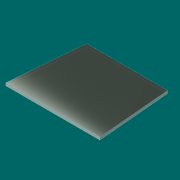
# Autodesk Inventor part: mirrorTopBottom
Saved by Autodesk Inventor 2016 (Build 200138000, 138)
## iProperties
Created: 2015-10-14
Part Number: mirrorTopBottom
Material: Glass
Document SubType Name: Modeling
Designer: Sawaiz
Density: 2.18 g/cm^3
Appearance: Clear
Author: Sawaiz
Autodesk Inventor part; units mm, degrees
ref_plane "YZ Plane" through (0, 0, 0) normal (1, 0, 0) x (0, 1, 0)
ref_plane "XZ Plane" through (0, 0, 0) normal (0, 1, 0) x (-1, 0, 0)
ref_plane "XY Plane" through (0, 0, 0) normal (0, 0, 1) x (1, 0, 0)
sketch "Sketch1" plane through (0, 0, 0) normal (0, 0, 1) x (1, 0, 0)
  line L0 (-37.1597, -43.7763) -> (-37.1597, 43.7763)
  line L1 (-37.1597, 43.7763) -> (43.1218, 50.8)
  line L2 (43.1218, 50.8) -> (43.1218, -50.8)
  line L3 (43.1218, -50.8) -> (-37.1597, -43.7763)
  line L4 (-37.1597, -43.7763) -> (43.1218, 50.8) construction
  line L5 (-37.1597, 43.7763) -> (43.1218, -50.8) construction
  point P0 (0, 0)
  dimension "d0" = 85
  dimension "d1" = 101.6
  dimension "d2" = 80.2815
  dimension "d5" = 87.5526
  constraints: 12 end point, 2 point on line, 1 equal length, 1 parallel, 1 vertical
  measures "d0" angle of L2 L1
  measures "d1" distance of L1.end L2.end
  measures "d2" distance between parallel lines of L2 L0
  measures "d5" distance of L0.start L0.end
extrude "Extrusion1" add sketch "Sketch1" along normal blind 3
equation "\"d1\" = width"
equation "\"d3\" = mirrorThickness"
equation "\"acrylicThickness\" = 6.35"
equation "\"height\" = 101.6"
equation "\"width\" = 101.6"
equation "\"depth\" = 101.6"
equation "\"mirrorAngle\" = 5deg"
equation "\"detectorWidth\" = 52"
equation "\"detectorHeight\" = 52"
equation "\"mirrorThickness\" = 3"
equation "\"fresnelThickness\" = 0.1"
equation "\"focalLength\" = 76.2"
equation "\"ior\" = 1.49"
equation "\"centerThickness\" = 1.524"
equation "\"fresnelAngle\" = 90deg"
equation "\"fresnelEffectiveDiameter\" = 76.2"
equation "\"mirrorSuppourtWidth\" = 38.1"
equation "\"sensorHolderORingID\" = 203.2"
equation "\"sensorHolderHeight\" = 88.9"
equation "\"oRingWidth\" = 3.175"
equation "\"sensorHolderSensorWidth\" = 53.975"
equation "\"sensorHolderFlushORingID\" = 254"
equation "\"sensorHolderWidth\" = 88.9"
equation "\"sensorHolderSensorHeight\" = 53.975"
equation "\"backGrooveBit\" = 4.8006"
equation "\"frontBackORingID\" = 419.1"
equation "\"mirrorGroove\" = 19.05"
equation "\"backMirrorGroove\" = 6.35"
equation "\"fresnelChamfer\" = 6.35"
equation "\"mirrorGrooveMill\" = 3.175"
body "Solid1"
